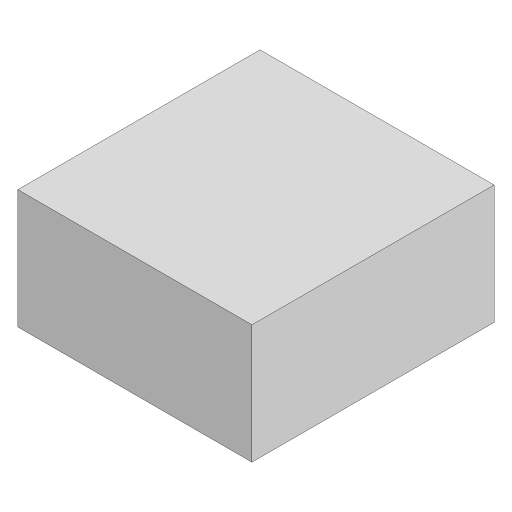
# Autodesk Inventor part: Part1
Saved by Autodesk Inventor 2024.2 (Build 282272000, 272)
## iProperties
Created: 2024-03-14
Part Number: Part1
Material: Generic
Document SubType Name: Modeling
Designer: Ilyas
Density: 1 g/cm^3
Appearance: Default
Author: Ilyas
Autodesk Inventor part; units mm, degrees
ref_plane "YZ Plane" through (0, 0, 0) normal (1, 0, 0) x (0, 1, 0)
ref_plane "XZ Plane" through (0, 0, 0) normal (0, 1, 0) x (-1, 0, 0)
ref_plane "XY Plane" through (0, 0, 0) normal (0, 0, 1) x (1, 0, 0)
sketch "Sketch1" plane through (0, 0, 0) normal (0, 0, 1) x (1, 0, 0)
  line L0 (-9.0946, -8.044) -> (10.5804, -8.044)
  line L1 (10.5804, -8.044) -> (10.5804, 12.3076)
  line L2 (10.5804, 12.3076) -> (-9.0946, 12.3076)
  line L3 (-9.0946, 12.3076) -> (-9.0946, -8.044)
  point P0 (0, 0)
  constraints: 8 end point, 2 parallel, 1 horizontal, 1 perpendicular
extrude "Extrusion1" add sketch "Sketch1" along normal blind 10
body "Solid1"
